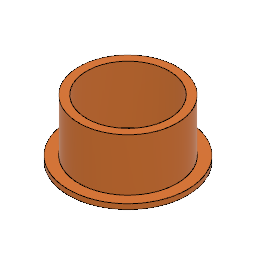
Guide feutre 3d (Autodesk Fusion 360 design; units mm, degrees)
Autodesk Fusion 360 part; units mm, degrees
sketch "Sketch tranche" plane through (0, 0, 0) normal (0, 0, 1) x (1, 0, 0)
  line L0 (0, 0) -> (1.5, 0)
  line L1 (1.5, 0) -> (1.5, 11)
  line L2 (1.5, 11) -> (0, 11)
  line L3 (0, 11) -> (0, 0)
  line L4 (-7.875, 0) -> (-7.875, 6)
  line L5 (1.5, 0) -> (3.5, 0)
  line L6 (3.5, 0) -> (3.5, 1)
  line L7 (3.5, 1) -> (1.5, 1)
  line L8 (1.5, 1) -> (1.5, 0)
  dimension "d1" = 11
  dimension "d2" = 1.5
  dimension "d3" = 7.875
  dimension "d5" = 2
  dimension "d6" = 1
  constraint horizontal L0
  constraint vertical L1
  constraint horizontal L2
  constraint vertical L3
  constraint coincident L0.start L3.end
  constraint vertical L4
  constraint horizontal L5
  constraint vertical L6
  constraint horizontal L7
  constraint vertical L8
  measures "d1" distance of L0.start L2.end
  measures "d2" distance of L0.start L0.end
  measures "d3" distance of L3 L4
  measures "d5" distance of L0.end L5.end
  measures "d6" distance of L0.end L7.end
revolve "Revolution tranche" add sketch "Sketch tranche" angle 360 about axis through (-7.875, 0, 0) along (0, 1, 0)
revolve "Revolve1" [suppressed]
named bodies: "tube", "Guide feutre"
